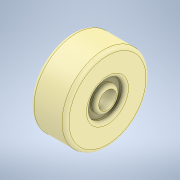
# Autodesk Inventor part: Rueda
Saved by Autodesk Inventor 2022.1 (Build 261234000, 234)
## iProperties
Created: 2021-09-11
Part Number: Rueda
Material: Genérico
Document SubType Name: Modeling
Designer: seb_0
Density: 1 g/cm^3
Appearance: Nilón 6
Author: seb_0
Autodesk Inventor part; units mm, degrees
ref_plane "YZ Plane" through (0, 0, 0) normal (1, 0, 0) x (0, 1, 0)
ref_plane "XZ Plane" through (0, 0, 0) normal (0, 1, 0) x (-1, 0, 0)
ref_plane "XY Plane" through (0, 0, 0) normal (0, 0, 1) x (1, 0, 0)
sketch "Boceto1" plane through (0, 0, 0) normal (1, 0, 0) x (0, 1, 0)
  circle A0 centre (0, 0) radius 60
  dimension "d0" = 120
  constraints: 1 centre point, 1 coincident
  measures "d0" diameter of A0
extrude "Extrusión1" add sketch "Boceto1" along normal blind 50
sketch "Boceto2" plane through (50, 0, 0) normal (1, 0, 0) x (0, 0, -1)
  circle A0 centre (0, 0) radius 25
  circle A1 centre (0, 0) radius 17.5
  dimension "d3" = 50
  dimension "d5" = 35
  constraints: 2 centre point, 2 coincident
  measures "d3" diameter of A0
  measures "d5" diameter of A1
fillet "Empalme1" radius 5 2 edges at (50, -60, 0) (0, -60, 0)
extrude "Extrusión2" cut sketch "Boceto2" against normal blind 7.5
fillet "Empalme2" radius 5 2 edges at (50, 0, 25) (50, 0, 17.5)
sketch "Boceto3" plane through (0, 0, 0) normal (-1, 0, 0) x (0, 0, 1)
  circle A0 centre (0, 0) radius 17.5 projected
  circle A1 centre (0, 0) radius 25 projected
extrude "Extrusión3" cut sketch "Boceto3" against normal blind 7.5
fillet "Empalme3" radius 5 2 edges at (0, 0, -25) (0, 0, -17.5)
sketch "Boceto4" plane through (50, 0, 0) normal (1, 0, 0) x (0, 0, -1)
  circle A0 centre (0, 0) radius 12.5 projected
extrude "Extrusión4" cut sketch "Boceto4" against normal through all
